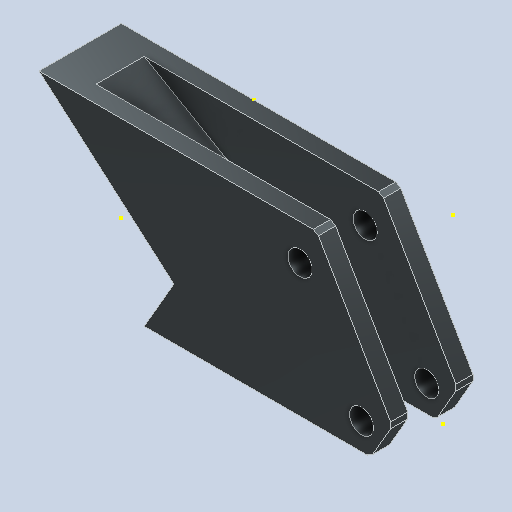
# Autodesk Inventor part: Non Colour Claw
Saved by Autodesk Inventor 2022 (Build 260153000, 153)
## iProperties
Created: 2021-06-22
Part Number: Non Colour Claw
Material: Iron, Gray
Document SubType Name: Modeling
Designer: Shreyas Darre
Density: 7.15 g/cm^3
Appearance: Iron Gray
Author: Shreyas Darre
Autodesk Inventor part; units mm, degrees
ref_plane "YZ Plane" through (0, 0, 0) normal (1, 0, 0) x (0, 1, 0)
ref_plane "XZ Plane" through (0, 0, 0) normal (0, 1, 0) x (-1, 0, 0)
ref_plane "XY Plane" through (0, 0, 0) normal (0, 0, 1) x (1, 0, 0)
sketch "Sketch2" plane through (0, 0, 0) normal (0, 0, 1) x (1, 0, 0)
  line L0 (0, 0) -> (51.3842, 0)
  line L1 (51.3842, 0) -> (65.3796, -24.2407)
  line L2 (65.3796, -24.2407) -> (61.3791, -31.1698)
  line L3 (65.3796, -24.2407) -> (73.3806, -24.2407) construction
  line L4 (61.3791, -31.1698) -> (19.4691, -31.1698)
  line L5 (19.4691, -31.1698) -> (24.9555, -21.6671)
  line L6 (19.4691, -31.1698) -> (30.4419, -31.1698) construction
  line L7 (24.9555, -21.6671) -> (0, 0)
  line L8 (51.3842, 0) -> (58.6918, 0) construction
  line L9 (48.8733, -7.5723) -> (70.4506, -7.5723) construction
  circle A0 centre (48.2959, -6.6229) radius 2.2225
  circle A1 centre (59.662, -26.2588) radius 2.2225
  dimension "d0" = 51.3842
  dimension "d1" = 27.9908
  dimension "d2" = 120
  dimension "d3" = 8.001
  dimension "d4" = 120
  dimension "d5" = 41.91
  dimension "d6" = 10.9728
  dimension "d7" = 60
  dimension "d15" = 4.445
  dimension "d16" = 4.445
  constraints: 20 end point, 6 horizontal, 2 centre point, 2 equal length
  measures "d0" distance of L0.start L0.end
  measures "d1" distance of L0.end L1.end
  measures "d2" angle of L0 L1
  measures "d3" distance of L1.end L2.end
  measures "d4" angle of L2 L3
  measures "d5" distance of L2.end L4.end
  measures "d6" distance of L4.end L5.end
  measures "d7" angle of L6 L5
  measures "d15" diameter of A0
  measures "d16" diameter of A1
extrude "Extrusion1" add sketch "Sketch2" along normal blind 15.24
sketch "Sketch3" plane through (65.3796, -24.2407, 15.24) normal (0.866, -0.5, 0) x (0, 0, -1)
  point P0 (15.24, -11.6967)
sketch "Sketch4" plane through (65.3796, -24.2407, 15.24) normal (0.866, -0.5, 0) x (0, 0, -1)
  line L0 (15.24, -8.001) -> (0, -8.001) projected
  line L1 (0, -8.001) -> (3.175, -8.001)
  line L2 (15.24, 0) -> (0, 0) projected
  line L3 (3.175, -8.001) -> (12.065, -8.001)
  line L4 (12.065, -8.001) -> (12.065, 0)
  line L5 (12.065, 0) -> (3.175, 0)
  line L6 (3.175, 0) -> (3.175, -8.001)
  point P0 (15.24, -11.6967)
  point P1 (3.175, 0)
  point P2 (12.065, -8.001)
  dimension "d19" = 3.175
  dimension "d20" = 8.89
  constraints: 10 end point, 2 parallel, 2 point on line, 1 horizontal, 1 perpendicular
  measures "d19" distance of L0.end L1.end
  measures "d20" distance of L5.end L4.end
sketch "Sketch5" plane through (19.4691, -31.1698, 0) normal (0, -1, 0) x (1, 0, 0)
  point P0 (-19.4691, 0)
extrude "Extrusion2" cut sketch "Sketch4" against normal blind 127
sketch "Sketch6" plane through (19.4691, -31.1698, 0) normal (0, -1, 0) x (1, 0, 0)
  point P0 (-19.4691, 0)
sketch "Sketch7" plane through (19.4691, -31.1698, 0) normal (0, -1, 0) x (1, 0, 0)
  line L0 (0, 0) -> (41.91, 0) projected
  line L1 (41.91, 3.175) -> (41.91, 12.065) projected
  line L2 (41.91, 0) -> (41.91, 3.175)
  line L3 (41.91, 12.065) -> (-12.0777, 12.065) projected
  line L4 (41.91, 3.175) -> (5.08, 3.175)
  line L5 (5.08, 12.065) -> (41.91, 12.065)
  line L6 (41.91, 12.065) -> (41.91, 3.175)
  line L7 (6.7536, 12.065) -> (6.7536, 3.175)
  line L8 (41.91, 3.175) -> (-12.0777, 3.175) projected
  point P0 (-19.4691, 0)
  dimension "d23" = 36.83
  constraints: 10 end point, 3 point on line, 1 collinear, 1 horizontal, 1 parallel, 1 vertical
  measures "d23" distance of L5.start L5.end
extrude "Extrusion3" [suppressed]
sketch "Sketch8" plane through (0, 0, 0) normal (0, 1, 0) x (1, 0, 0)
  line L0 (65.3796, -3.175) -> (23.3934, -3.175) projected
  line L1 (24.5491, -3.175) -> (23.3934, -3.175)
  line L2 (23.3934, -12.065) -> (7.3914, -12.065) projected
  line L3 (24.5491, -3.175) -> (23.3934, -3.175)
  line L4 (23.3934, -3.175) -> (23.3934, -12.065)
  line L5 (23.3934, -12.065) -> (24.5491, -12.065)
  line L6 (24.5491, -12.065) -> (24.5491, -3.175)
  point P0 (0, 0)
  constraints: 10 end point, 2 parallel, 1 collinear, 1 horizontal, 1 perpendicular
extrude "Extrusion4" cut sketch "Sketch8" along normal mid plane 15.24
sketch "Sketch9" plane through (61.3791, -21.9311, 3.175) normal (-1, 0, 0) x (0, 0, 1)
  point P0 (-3.175, 21.9311)
sketch "Sketch10" plane through (65.3796, -24.2407, 12.065) normal (0.866, 0.5, 0) x (0, 0, -1)
  line L0 (8.89, 0) -> (0, 0) projected
  line L1 (8.89, 4.0005) -> (8.89, 8.001) projected
  line L2 (0, 0) -> (8.89, 0)
  line L3 (8.89, 0) -> (8.89, 8.001)
  line L4 (8.89, 8.001) -> (0, 8.001)
  line L5 (0, 8.001) -> (0, 0)
  point P0 (12.065, 53.6829)
  constraints: 8 end point, 2 parallel, 1 horizontal, 1 perpendicular
extrude "Extrusion5" cut sketch "Sketch10" against normal blind 15.24
sketch "Sketch11" plane through (19.4691, -31.1698, 0) normal (0, -1, 0) x (1, 0, 0)
  line L0 (42.4154, 3.175) -> (37.9704, 3.175) projected
  line L1 (42.4154, 3.175) -> (6.2959, 3.175)
  line L2 (6.2959, 3.175) -> (6.2959, 12.065)
  line L3 (6.2959, 12.065) -> (42.4154, 12.065)
  line L4 (42.4154, 12.065) -> (42.4154, 3.175)
  point P0 (-19.4691, 0)
  constraints: 8 end point, 2 parallel, 1 horizontal, 1 perpendicular
extrude "Extrusion6" cut sketch "Sketch11" against normal blind 127
sketch "Sketch12" plane through (24.5491, 0, 3.175) normal (-1, 0, 0) x (0, 0, 1)
  point P0 (-3.175, 0)
sketch "Sketch13" plane through (0, 0, 0) normal (0, 1, 0) x (1, 0, 0)
  line L0 (25.765, -3.175) -> (24.5491, -3.175) projected
  line L1 (25.765, -3.175) -> (25.765, -12.065) projected
  line L2 (24.5491, -3.175) -> (25.765, -3.175)
  line L3 (25.765, -3.175) -> (25.765, -12.065)
  line L4 (25.765, -12.065) -> (24.5491, -12.065)
  line L5 (24.5491, -12.065) -> (24.5491, -3.175)
  point P0 (0, 0)
  constraints: 8 end point, 2 parallel, 1 horizontal, 1 perpendicular
extrude "Extrusion7" cut sketch "Sketch13" against normal blind 2.54
chamfer "Chamfer1" distance 0.635 angle 45 6 edges at (61.3791, -31.1698, 13.6525) (65.3796, -24.2407, 13.6525) (65.3796, -24.2407, 1.5875) (61.3791, -31.1698, 1.5875) (51.3842, 0, 13.6525) (51.3842, 0, 1.5875)
body "Solid1"
